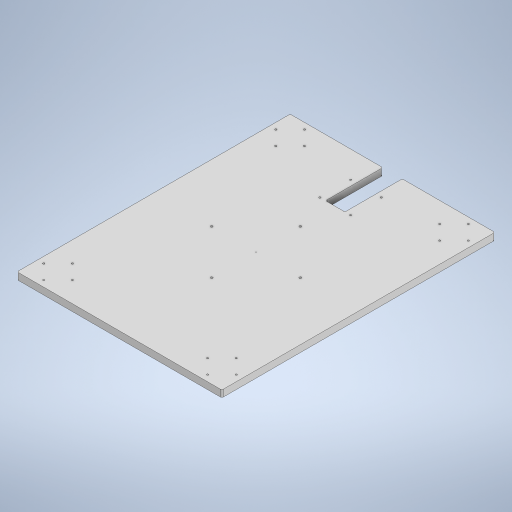
# Autodesk Inventor part: turntablebase
Saved by Autodesk Inventor 2024 (Build 280153000, 153)
## iProperties
Created: 2023-09-10
Part Number: turntablebase
Material: Generic
Document SubType Name: Modeling
Designer: Wei Ting
Density: 1 g/cm^3
Appearance: Default
Author: Wei Ting
Autodesk Inventor part; units mm, degrees
ref_plane "YZ Plane" through (0, 0, 0) normal (1, 0, 0) x (0, 1, 0)
ref_plane "XZ Plane" through (0, 0, 0) normal (0, 1, 0) x (-1, 0, 0)
ref_plane "XY Plane" through (0, 0, 0) normal (0, 0, 1) x (1, 0, 0)
sketch "Sketch1" plane through (0, 0, 0) normal (0, 1, 0) x (-1, 0, 0)
  line L0 (300, 400) -> (-300, 400)
  line L1 (-300, 400) -> (-300, -400)
  line L2 (-300, -400) -> (300, -400)
  line L3 (300, -400) -> (300, 400)
  line L4 (300, 400) -> (-300, -400) construction
  circle A0 centre (130, 0) radius 3
  circle A1 centre (0, 130) radius 3
  circle A2 centre (-130, 0) radius 3
  circle A3 centre (0, -130) radius 3
  circle A4 centre (0, 0) radius 277.128
  line L5 (45, -232.128) -> (-45, -232.128)
  line L6 (-45, -232.128) -> (-45, -322.128)
  line L7 (-45, -322.128) -> (45, -322.128)
  line L8 (45, -322.128) -> (45, -232.128)
  line L9 (45, -232.128) -> (-45, -322.128) construction
  line L10 (-45, -232.128) -> (45, -322.128) construction
  circle A5 centre (45, -232.128) radius 2.5
  line L11 (28.5, -232.128) -> (-28.5, -232.128)
  line L12 (-28.5, -232.128) -> (-28.5, -322.128)
  line L13 (-28.5, -322.128) -> (28.5, -322.128)
  line L14 (28.5, -322.128) -> (28.5, -232.128)
  line L15 (28.5, -232.128) -> (-28.5, -322.128) construction
  line L16 (-28.5, -232.128) -> (28.5, -322.128) construction
  line L17 (45, -322.128) -> (-45, -322.128)
  line L18 (-45, -322.128) -> (-45, -400)
  line L19 (-45, -400) -> (45, -400)
  line L20 (45, -400) -> (45, -322.128)
  line L21 (28.5, -322.128) -> (-28.5, -322.128)
  line L22 (-28.5, -322.128) -> (-28.5, -400)
  line L23 (-28.5, -400) -> (28.5, -400)
  line L24 (28.5, -400) -> (28.5, -322.128)
  circle A6 centre (45, -322.128) radius 2.5
  circle A7 centre (-45, -232.128) radius 2.5
  circle A8 centre (-45, -322.128) radius 2.5
  circle A9 centre (0, 0) radius 1
  point P0 (0, -277.128)
  point P1 (28.5, -400)
  dimension "d10" = 554.256
  dimension "d0" = 600
  dimension "d1" = 800
  dimension "d2" = 6
  dimension "d3" = 130
  dimension "d6" = 360
  dimension "d41" = 90
  dimension "d42" = 90
  dimension "d43" = 5
  dimension "d52" = 57
  dimension "d75" = 90
  dimension "d78" = 90
  dimension "d82" = 2
  constraints: 50 end point, 10 parallel, 9 centre point, 6 horizontal, 5 midpoint, 5 perpendicular, 3 coincident, 3 point on line, 1 vertical, 1 vertical alignment, 17 other
  measures "d0" distance of L2.end L1.end
  measures "d1" distance of L0.end L1.end
  measures "d2" diameter of A0
  measures "d3" distance of point (0, 0) A0.centre
  measures "d41" distance of L6.end L7.end
  measures "d42" distance of L5.end L6.end
  measures "d43" diameter of A5
  measures "d52" distance between parallel lines of L12 L14
  measures "d75" distance of A5.centre A6.centre
  measures "d78" distance of A5.centre A7.centre
  measures "d82" diameter of A9
extrude "Extrusion1" add sketch "Sketch1" along normal blind 20 contours L3 L2 L20 A6 L8 A4 L6 A8 L18 L1 L0 | L2 L24 L7 A6 L20 | L18 A8 L7 L22 L2 | L14 A4 L8 A6 L7 | L7 A8 L6 A4 L12 | L14 L5 A5 L8 A4 | A4 L6 A7 L5 L12 | A4 L8 A5 L5 A7 L6
sketch "Sketch3" plane through (0, 20, 0) normal (0, 1, 0) x (1, 0, 0)
  line L0 (-300, -400) -> (-180, -400)
  line L1 (-180, -400) -> (-180, -280)
  line L2 (-180, -280) -> (-300, -280)
  line L3 (-300, -280) -> (-300, -400)
  line L4 (-300, -400) -> (-180, -280) construction
  line L5 (-180, -400) -> (-300, -280) construction
  line L6 (-300, 400) -> (-300, -400) projected
  line L7 (-300, -400) -> (300, -400) projected
  circle A0 centre (-282, -340) radius 2.5
  circle A1 centre (-240, -382) radius 2.5
  circle A2 centre (-198, -340) radius 2.5
  circle A3 centre (-240, -298) radius 2.5
  line L8 (300, 400) -> (-300, 400) projected
  circle A4 centre (-240, 382) radius 2.5
  line L9 (-300, 400) -> (-300, 280)
  line L10 (-180, 280) -> (-300, 400) construction
  line L11 (-180, 280) -> (-180, 400)
  line L12 (-180, 400) -> (-300, 400)
  line L13 (-300, 280) -> (-180, 400) construction
  circle A5 centre (-198, 340) radius 2.5
  circle A6 centre (-282, 340) radius 2.5
  circle A7 centre (-240, 298) radius 2.5
  line L14 (-300, 280) -> (-180, 280)
  circle A8 centre (240, -298) radius 2.5
  line L15 (180, -280) -> (180, -400)
  line L16 (300, -400) -> (180, -280) construction
  line L17 (300, -400) -> (300, -280)
  line L18 (300, -280) -> (180, -280)
  line L19 (180, -400) -> (300, -280) construction
  circle A9 centre (282, -340) radius 2.5
  circle A10 centre (198, -340) radius 2.5
  circle A11 centre (240, -382) radius 2.5
  line L20 (180, -400) -> (300, -400)
  circle A12 centre (240, 382) radius 2.5
  line L21 (180, 400) -> (180, 280)
  line L22 (300, 280) -> (180, 400) construction
  line L23 (300, 280) -> (300, 400)
  line L24 (300, 400) -> (180, 400)
  line L25 (180, 280) -> (300, 400) construction
  circle A13 centre (282, 340) radius 2.5
  circle A14 centre (198, 340) radius 2.5
  circle A15 centre (240, 298) radius 2.5
  line L26 (180, 280) -> (300, 280)
  point P0 (0, 0)
  point P1 (-240, -340)
  point P2 (-240, 340)
  point P3 (240, -340)
  point P4 (240, 340)
  dimension "d53" = 120
  dimension "d54" = 120
  dimension "d55" = 60
  dimension "d56" = 60
  dimension "d57" = 5
  dimension "d58" = 42
  dimension "d61" = 360
  dimension "d67" = 680
  dimension "d70" = 480
  constraints: 48 end point, 16 centre point, 2 horizontal, 2 midpoint, 2 parallel, 1 perpendicular, 1 vertical, 66 other
  measures "d53" distance of L1.end L2.end
  measures "d54" distance of L0.end L1.end
  measures "d55" distance from line of L6 point (-240, -340)
  measures "d56" distance from line of L7 point (-240, -340)
  measures "d57" diameter of A0
  measures "d58" distance of A0.centre point (-240, -340)
  measures "d67" distance of A3.centre A4.centre
  measures "d70" distance of A3.centre A8.centre
extrude "Extrusion3" cut sketch "Sketch3" against normal through all contours A0 | A1 | A2 | A3 | A4 | A5 | A6 | A7 | A8 | A9 | A10 | A11 | A12 | A13 | A14 | A15
fillet "Fillet3" radius 5 8 edges at (300, 10, 400) (300, 10, -400) (-28.5, 10, -400) (28.5, 10, -400) (-28.5, 10, -232.128) (28.5, 10, -232.128) (-300, 10, -400) (-300, 10, 400)
equation "\"d0\" = Width"
equation "\"d1\" = Length"
equation "\"d3\" = BearingHoleRadius1"
equation "\"Width\" = 600"
equation "\"Length\" = 800"
equation "\"BearingHoleRadius1\" = 130"
body "Solid1"
